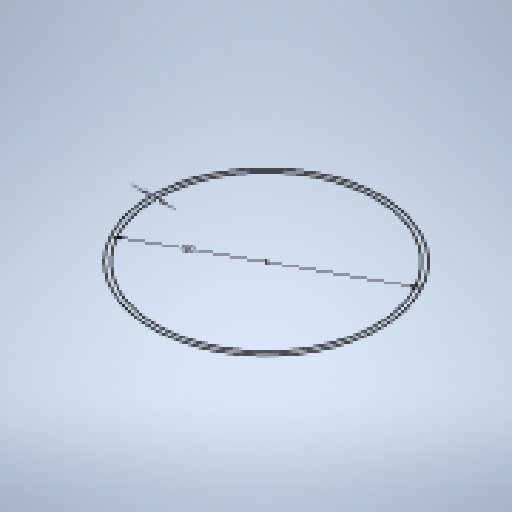
# Autodesk Inventor part: Dummy 3
Saved by Autodesk Inventor 2025 (Build 290162010, 162A)
## iProperties
Created: 2024-07-24
Part Number: Dummy 3
Material: Generic
Document SubType Name: Modeling
Designer: admin
Density: 1 g/cm^3
Appearance: Default
Author: admin
Autodesk Inventor part; units mm, degrees
ref_plane "YZ Plane" through (0, 0, 0) normal (1, 0, 0) x (0, 1, 0)
ref_plane "XZ Plane" through (0, 0, 0) normal (0, 1, 0) x (-1, 0, 0)
ref_plane "XY Plane" through (0, 0, 0) normal (0, 0, 1) x (1, 0, 0)
sketch "Sketch1" plane through (0, 0, 0) normal (0, 0, 1) x (1, 0, 0)
  circle A0 centre (0, 0) radius 25
  circle A1 centre (0, 0) radius 24
  dimension "d0" = 50
  dimension "d1" = 1
  constraints: 2 centre point, 1 coincident
  measures "d0" diameter of A0
  measures "d1" radial gap between concentric circles of A0 A1
extrude "Extrusion1" add sketch "Sketch1" along normal blind 1000
sketch "Sketch2" plane through (0, 0, 0) normal (0, 1, 0) x (-1, 0, 0)
  line L0 (-1.5, 5.4) -> (1.5, 5.4)
  line L1 (1.5, 5.4) -> (1.5, 5)
  line L2 (1.5, 5) -> (-1.5, 5)
  line L3 (-1.5, 5) -> (-1.5, 5.4)
  point P0 (0, 0)
  point P1 (0, 5)
  dimension "d4" = 3
  dimension "d5" = 0.4
  dimension "d6" = 5
  constraints: 8 end point, 2 parallel, 1 horizontal, 1 midpoint, 1 perpendicular, 1 vertical alignment
  measures "d4" distance of L1.end L2.end
  measures "d5" distance of L0.end L1.end
  measures "d6" distance from line of point (0, 0) L2
extrude "Extrusion2" cut sketch "Sketch2" against normal through all
pattern_circular "Circular Pattern1" count 12 over 180 about axis through (0, 0, 0) along (0, 0, 1) of "Extrusion2" both ways yes
pattern_linear "Rectangular Pattern1" count 10 spacing 5 along (0, 0, 1) of "Extrusion2", "Circular Pattern1"
body "Solid1"
